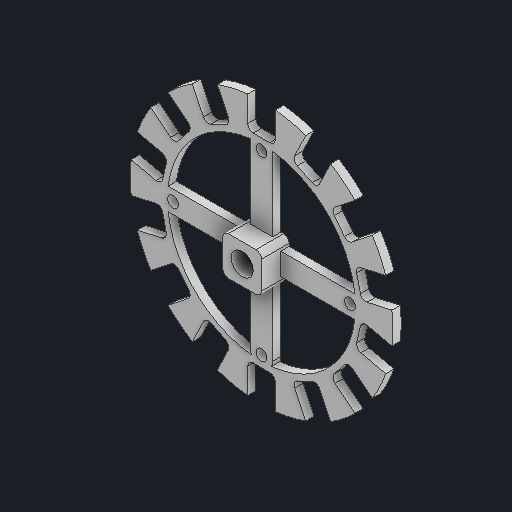
# Autodesk Inventor part: OmniFrame_A
Saved by Autodesk Inventor 2024.2 (Build 282272000, 272)
## iProperties
Created: 2023-12-20
Part Number: OmniFrame_A
Material: 一般
Document SubType Name: Modeling
Designer: Hanaoka
Density: 1 g/cm^3
Appearance: 既定
Author: Hanaoka
Autodesk Inventor part; units mm, degrees
ref_plane "YZ Plane" through (0, 0, 0) normal (1, 0, 0) x (0, 1, 0)
ref_plane "XZ Plane" through (0, 0, 0) normal (0, 1, 0) x (-1, 0, 0)
ref_plane "XY Plane" through (0, 0, 0) normal (0, 0, 1) x (1, 0, 0)
derived "OmniFrame_B.ipt"
sketch "スケッチ1" plane through (0, 0, 0) normal (0, 0, 1) x (1, 0, 0)
  circle A0 centre (0, 0) radius 25 construction
  line L0 (-2.5, 24.8747) -> (-2.5, 19)
  line L1 (-1.5, 18) -> (1.5, 18)
  line L2 (2.5, 19) -> (2.5, 24.8747)
  line L3 (0, 25) -> (0, 18) construction
  line L4 (-2.5, 23.025) -> (-3, 23.025)
  line L5 (-4, 22.025) -> (-4, 21.975)
  line L6 (-3, 20.975) -> (-2.5, 20.975)
  line L7 (2.5, 23.025) -> (3, 23.025)
  line L8 (4, 22.025) -> (4, 21.975)
  line L9 (3, 20.975) -> (2.5, 20.975)
  arc A1 (-3, 23.025) -> (-4, 22.025) centre (-3, 22.025) ccw
  arc A2 (-4, 21.975) -> (-3, 20.975) centre (-3, 21.975) ccw
  arc A3 (4, 22.025) -> (3, 23.025) centre (3, 22.025) ccw
  arc A4 (3, 20.975) -> (4, 21.975) centre (3, 21.975) ccw
  arc A5 (-2.5, 19) -> (-1.5, 18) centre (-1.5, 19) ccw
  arc A6 (1.5, 18) -> (2.5, 19) centre (1.5, 19) ccw
  arc A7 (-10.4962, 16.0337) -> (-9.1614, 15.5666) centre (-9.5952, 16.4676) ccw
  arc A8 (-6.4585, 16.8683) -> (-5.9914, 18.2031) centre (-6.8923, 17.7692) ccw
  line L10 (-9.1614, 15.5666) -> (-6.4585, 16.8683)
  line L11 (-6.3978, 20.1995) -> (-6.8483, 19.9825)
  arc A9 (-6.3978, 20.1995) -> (-5.9307, 21.5343) centre (-6.8317, 21.1004) ccw
  line L12 (-5.9524, 21.5794) -> (-5.9307, 21.5343)
  arc A10 (-5.9524, 21.5794) -> (-7.2873, 22.0465) centre (-6.8534, 21.1455) ccw
  line L13 (-7.7378, 21.8295) -> (-7.2873, 22.0465)
  line L14 (-11.8036, 17.5962) -> (-11.3531, 17.8131)
  line L15 (-5.9914, 18.2031) -> (-8.5403, 23.496)
  line L16 (-10.8471, 22.5242) -> (-7.8099, 16.2174) construction
  line L17 (-13.0451, 21.3266) -> (-10.4962, 16.0337)
  arc A11 (-13.1385, 18.0633) -> (-11.8036, 17.5962) centre (-12.2375, 18.4971) ccw
  line L18 (-12.2426, 19.6601) -> (-12.6931, 19.4432)
  line L19 (-13.1602, 18.1083) -> (-13.1385, 18.0633)
  arc A12 (-12.6931, 19.4432) -> (-13.1602, 18.1083) centre (-12.2592, 18.5422) ccw
  arc A13 (-16.4135, 9.8917) -> (-15.0082, 10.0501) centre (-15.79, 10.6736) ccw
  arc A14 (-13.1377, 12.3956) -> (-13.2961, 13.8009) centre (-13.9196, 13.0191) ccw
  line L20 (-15.0082, 10.0501) -> (-13.1377, 12.3956)
  line L21 (-14.5284, 15.4232) -> (-14.8402, 15.0323)
  arc A15 (-14.5284, 15.4232) -> (-14.6868, 16.8285) centre (-15.3103, 16.0467) ccw
  line L22 (-14.7259, 16.8597) -> (-14.6868, 16.8285)
  arc A16 (-14.7259, 16.8597) -> (-16.1312, 16.7013) centre (-15.3494, 16.0779) ccw
  line L23 (-16.4429, 16.3104) -> (-16.1312, 16.7013)
  line L24 (-18.2694, 10.7322) -> (-17.9576, 11.1231)
  line L25 (-13.2961, 13.8009) -> (-17.8891, 17.4637)
  line L26 (-19.5458, 15.5872) -> (-14.073, 11.2228) construction
  line L27 (-21.0065, 13.5545) -> (-16.4135, 9.8917)
  arc A17 (-19.6747, 10.5739) -> (-18.2694, 10.7322) centre (-19.0512, 11.3557) ccw
  line L28 (-19.5604, 12.4013) -> (-19.8721, 12.0104)
  line L29 (-19.7138, 10.605) -> (-19.6747, 10.5739)
  arc A18 (-19.8721, 12.0104) -> (-19.7138, 10.605) centre (-19.0903, 11.3869) ccw
  arc A19 (-19.0799, 1.7906) -> (-17.8825, 2.543) centre (-18.8574, 2.7655) ccw
  arc A20 (-17.2149, 5.4678) -> (-17.9673, 6.6652) centre (-18.1898, 5.6903) ccw
  line L30 (-17.8825, 2.543) -> (-17.2149, 5.4678)
  line L31 (-19.7816, 7.5922) -> (-19.8928, 7.1047)
  arc A21 (-19.7816, 7.5922) -> (-20.534, 8.7896) centre (-20.7565, 7.8147) ccw
  line L32 (-20.5827, 8.8007) -> (-20.534, 8.7896)
  arc A22 (-20.5827, 8.8007) -> (-21.7802, 8.0483) centre (-20.8052, 7.8258) ccw
  line L33 (-21.8914, 7.5609) -> (-21.7802, 8.0483)
  line L34 (-21.1167, 1.7426) -> (-21.0054, 2.2301)
  line L35 (-17.9673, 6.6652) -> (-23.6947, 7.9725)
  line L36 (-24.3732, 5.563) -> (-17.5487, 4.0054) construction
  line L37 (-24.8073, 3.0978) -> (-19.0799, 1.7906)
  arc A23 (-22.3141, 0.9902) -> (-21.1167, 1.7426) centre (-22.0916, 1.9651) ccw
  line L38 (-23.004, 2.6862) -> (-23.1153, 2.1988)
  line L39 (-22.3629, 1.0013) -> (-22.3141, 0.9902)
  arc A24 (-23.1153, 2.1988) -> (-22.3629, 1.0013) centre (-22.1404, 1.9762) ccw
  arc A25 (-17.9673, -6.6652) -> (-17.2149, -5.4678) centre (-18.1898, -5.6903) ccw
  arc A26 (-17.8825, -2.543) -> (-19.0799, -1.7906) centre (-18.8574, -2.7655) ccw
  line L40 (-17.2149, -5.4678) -> (-17.8825, -2.543)
  line L41 (-21.1167, -1.7426) -> (-21.0054, -2.2301)
  arc A27 (-21.1167, -1.7426) -> (-22.3141, -0.9902) centre (-22.0916, -1.9651) ccw
  line L42 (-22.3629, -1.0013) -> (-22.3141, -0.9902)
  arc A28 (-22.3629, -1.0013) -> (-23.1153, -2.1988) centre (-22.1404, -1.9762) ccw
  line L43 (-23.004, -2.6862) -> (-23.1153, -2.1988)
  line L44 (-19.7816, -7.5922) -> (-19.8928, -7.1047)
  line L45 (-19.0799, -1.7906) -> (-24.8073, -3.0978)
  line L46 (-24.3732, -5.563) -> (-17.5487, -4.0054) construction
  line L47 (-23.6947, -7.9725) -> (-17.9673, -6.6652)
  arc A29 (-20.534, -8.7896) -> (-19.7816, -7.5922) centre (-20.7565, -7.8147) ccw
  line L48 (-21.8914, -7.5609) -> (-21.7802, -8.0483)
  line L49 (-20.5827, -8.8007) -> (-20.534, -8.7896)
  arc A30 (-21.7802, -8.0483) -> (-20.5827, -8.8007) centre (-20.8052, -7.8258) ccw
  arc A31 (-13.2961, -13.8009) -> (-13.1377, -12.3956) centre (-13.9196, -13.0191) ccw
  arc A32 (-15.0082, -10.0501) -> (-16.4135, -9.8917) centre (-15.79, -10.6736) ccw
  line L50 (-13.1377, -12.3956) -> (-15.0082, -10.0501)
  line L51 (-18.2694, -10.7322) -> (-17.9576, -11.1231)
  arc A33 (-18.2694, -10.7322) -> (-19.6747, -10.5739) centre (-19.0512, -11.3557) ccw
  line L52 (-19.7138, -10.605) -> (-19.6747, -10.5739)
  arc A34 (-19.7138, -10.605) -> (-19.8721, -12.0104) centre (-19.0903, -11.3869) ccw
  line L53 (-19.5604, -12.4013) -> (-19.8721, -12.0104)
  line L54 (-14.5284, -15.4232) -> (-14.8402, -15.0323)
  line L55 (-16.4135, -9.8917) -> (-21.0065, -13.5545)
  line L56 (-19.5458, -15.5872) -> (-14.073, -11.2228) construction
  line L57 (-17.8891, -17.4637) -> (-13.2961, -13.8009)
  arc A35 (-14.6868, -16.8285) -> (-14.5284, -15.4232) centre (-15.3103, -16.0467) ccw
  line L58 (-16.4429, -16.3104) -> (-16.1312, -16.7013)
  line L59 (-14.7259, -16.8597) -> (-14.6868, -16.8285)
  arc A36 (-16.1312, -16.7013) -> (-14.7259, -16.8597) centre (-15.3494, -16.0779) ccw
  arc A37 (-5.9914, -18.2031) -> (-6.4585, -16.8683) centre (-6.8923, -17.7692) ccw
  arc A38 (-9.1614, -15.5666) -> (-10.4962, -16.0337) centre (-9.5952, -16.4676) ccw
  line L60 (-6.4585, -16.8683) -> (-9.1614, -15.5666)
  line L61 (-11.8036, -17.5962) -> (-11.3531, -17.8131)
  arc A39 (-11.8036, -17.5962) -> (-13.1385, -18.0633) centre (-12.2375, -18.4971) ccw
  line L62 (-13.1602, -18.1083) -> (-13.1385, -18.0633)
  arc A40 (-13.1602, -18.1083) -> (-12.6931, -19.4432) centre (-12.2592, -18.5422) ccw
  line L63 (-12.2426, -19.6601) -> (-12.6931, -19.4432)
  line L64 (-6.3978, -20.1995) -> (-6.8483, -19.9825)
  line L65 (-10.4962, -16.0337) -> (-13.0451, -21.3266)
  line L66 (-10.8471, -22.5242) -> (-7.8099, -16.2174) construction
  line L67 (-8.5403, -23.496) -> (-5.9914, -18.2031)
  arc A41 (-5.9307, -21.5343) -> (-6.3978, -20.1995) centre (-6.8317, -21.1004) ccw
  line L68 (-7.7378, -21.8295) -> (-7.2873, -22.0465)
  line L69 (-5.9524, -21.5794) -> (-5.9307, -21.5343)
  arc A42 (-7.2873, -22.0465) -> (-5.9524, -21.5794) centre (-6.8534, -21.1455) ccw
  arc A43 (2.5, -19) -> (1.5, -18) centre (1.5, -19) ccw
  arc A44 (-1.5, -18) -> (-2.5, -19) centre (-1.5, -19) ccw
  line L70 (1.5, -18) -> (-1.5, -18)
  line L71 (-3, -20.975) -> (-2.5, -20.975)
  arc A45 (-3, -20.975) -> (-4, -21.975) centre (-3, -21.975) ccw
  line L72 (-4, -22.025) -> (-4, -21.975)
  arc A46 (-4, -22.025) -> (-3, -23.025) centre (-3, -22.025) ccw
  line L73 (-2.5, -23.025) -> (-3, -23.025)
  line L74 (3, -20.975) -> (2.5, -20.975)
  line L75 (-2.5, -19) -> (-2.5, -24.8747)
  line L76 (0, -25) -> (0, -18) construction
  line L77 (2.5, -24.8747) -> (2.5, -19)
  arc A47 (4, -21.975) -> (3, -20.975) centre (3, -21.975) ccw
  line L78 (2.5, -23.025) -> (3, -23.025)
  line L79 (4, -22.025) -> (4, -21.975)
  arc A48 (3, -23.025) -> (4, -22.025) centre (3, -22.025) ccw
  arc A49 (10.4962, -16.0337) -> (9.1614, -15.5666) centre (9.5952, -16.4676) ccw
  arc A50 (6.4585, -16.8683) -> (5.9914, -18.2031) centre (6.8923, -17.7692) ccw
  line L80 (9.1614, -15.5666) -> (6.4585, -16.8683)
  line L81 (6.3978, -20.1995) -> (6.8483, -19.9825)
  arc A51 (6.3978, -20.1995) -> (5.9307, -21.5343) centre (6.8317, -21.1004) ccw
  line L82 (5.9524, -21.5794) -> (5.9307, -21.5343)
  arc A52 (5.9524, -21.5794) -> (7.2873, -22.0465) centre (6.8534, -21.1455) ccw
  line L83 (7.7378, -21.8295) -> (7.2873, -22.0465)
  line L84 (11.8036, -17.5962) -> (11.3531, -17.8131)
  line L85 (5.9914, -18.2031) -> (8.5403, -23.496)
  line L86 (10.8471, -22.5242) -> (7.8099, -16.2174) construction
  line L87 (13.0451, -21.3266) -> (10.4962, -16.0337)
  arc A53 (13.1385, -18.0633) -> (11.8036, -17.5962) centre (12.2375, -18.4971) ccw
  line L88 (12.2426, -19.6601) -> (12.6931, -19.4432)
  line L89 (13.1602, -18.1083) -> (13.1385, -18.0633)
  arc A54 (12.6931, -19.4432) -> (13.1602, -18.1083) centre (12.2592, -18.5422) ccw
  arc A55 (16.4135, -9.8917) -> (15.0082, -10.0501) centre (15.79, -10.6736) ccw
  arc A56 (13.1377, -12.3956) -> (13.2961, -13.8009) centre (13.9196, -13.0191) ccw
  line L90 (15.0082, -10.0501) -> (13.1377, -12.3956)
  line L91 (14.5284, -15.4232) -> (14.8402, -15.0323)
  arc A57 (14.5284, -15.4232) -> (14.6868, -16.8285) centre (15.3103, -16.0467) ccw
  line L92 (14.7259, -16.8597) -> (14.6868, -16.8285)
  arc A58 (14.7259, -16.8597) -> (16.1312, -16.7013) centre (15.3494, -16.0779) ccw
  line L93 (16.4429, -16.3104) -> (16.1312, -16.7013)
  line L94 (18.2694, -10.7322) -> (17.9576, -11.1231)
  line L95 (13.2961, -13.8009) -> (17.8891, -17.4637)
  line L96 (19.5458, -15.5872) -> (14.073, -11.2228) construction
  line L97 (21.0065, -13.5545) -> (16.4135, -9.8917)
  arc A59 (19.6747, -10.5739) -> (18.2694, -10.7322) centre (19.0512, -11.3557) ccw
  line L98 (19.5604, -12.4013) -> (19.8721, -12.0104)
  line L99 (19.7138, -10.605) -> (19.6747, -10.5739)
  arc A60 (19.8721, -12.0104) -> (19.7138, -10.605) centre (19.0903, -11.3869) ccw
  arc A61 (19.0799, -1.7906) -> (17.8825, -2.543) centre (18.8574, -2.7655) ccw
  arc A62 (17.2149, -5.4678) -> (17.9673, -6.6652) centre (18.1898, -5.6903) ccw
  line L100 (17.8825, -2.543) -> (17.2149, -5.4678)
  line L101 (19.7816, -7.5922) -> (19.8928, -7.1047)
  arc A63 (19.7816, -7.5922) -> (20.534, -8.7896) centre (20.7565, -7.8147) ccw
  line L102 (20.5827, -8.8007) -> (20.534, -8.7896)
  arc A64 (20.5827, -8.8007) -> (21.7802, -8.0483) centre (20.8052, -7.8258) ccw
  line L103 (21.8914, -7.5609) -> (21.7802, -8.0483)
  line L104 (21.1167, -1.7426) -> (21.0054, -2.2301)
  line L105 (17.9673, -6.6652) -> (23.6947, -7.9725)
  line L106 (24.3732, -5.563) -> (17.5487, -4.0054) construction
  line L107 (24.8073, -3.0978) -> (19.0799, -1.7906)
  arc A65 (22.3141, -0.9902) -> (21.1167, -1.7426) centre (22.0916, -1.9651) ccw
  line L108 (23.004, -2.6862) -> (23.1153, -2.1988)
  line L109 (22.3629, -1.0013) -> (22.3141, -0.9902)
  arc A66 (23.1153, -2.1988) -> (22.3629, -1.0013) centre (22.1404, -1.9762) ccw
  arc A67 (17.9673, 6.6652) -> (17.2149, 5.4678) centre (18.1898, 5.6903) ccw
  arc A68 (17.8825, 2.543) -> (19.0799, 1.7906) centre (18.8574, 2.7655) ccw
  line L110 (17.2149, 5.4678) -> (17.8825, 2.543)
  line L111 (21.1167, 1.7426) -> (21.0054, 2.2301)
  arc A69 (21.1167, 1.7426) -> (22.3141, 0.9902) centre (22.0916, 1.9651) ccw
  line L112 (22.3629, 1.0013) -> (22.3141, 0.9902)
  arc A70 (22.3629, 1.0013) -> (23.1153, 2.1988) centre (22.1404, 1.9762) ccw
  line L113 (23.004, 2.6862) -> (23.1153, 2.1988)
  line L114 (19.7816, 7.5922) -> (19.8928, 7.1047)
  line L115 (19.0799, 1.7906) -> (24.8073, 3.0978)
  line L116 (24.3732, 5.563) -> (17.5487, 4.0054) construction
  line L117 (23.6947, 7.9725) -> (17.9673, 6.6652)
  arc A71 (20.534, 8.7896) -> (19.7816, 7.5922) centre (20.7565, 7.8147) ccw
  line L118 (21.8914, 7.5609) -> (21.7802, 8.0483)
  line L119 (20.5827, 8.8007) -> (20.534, 8.7896)
  arc A72 (21.7802, 8.0483) -> (20.5827, 8.8007) centre (20.8052, 7.8258) ccw
  arc A73 (13.2961, 13.8009) -> (13.1377, 12.3956) centre (13.9196, 13.0191) ccw
  arc A74 (15.0082, 10.0501) -> (16.4135, 9.8917) centre (15.79, 10.6736) ccw
  line L120 (13.1377, 12.3956) -> (15.0082, 10.0501)
  line L121 (18.2694, 10.7322) -> (17.9576, 11.1231)
  arc A75 (18.2694, 10.7322) -> (19.6747, 10.5739) centre (19.0512, 11.3557) ccw
  line L122 (19.7138, 10.605) -> (19.6747, 10.5739)
  arc A76 (19.7138, 10.605) -> (19.8721, 12.0104) centre (19.0903, 11.3869) ccw
  line L123 (19.5604, 12.4013) -> (19.8721, 12.0104)
  line L124 (14.5284, 15.4232) -> (14.8402, 15.0323)
  line L125 (16.4135, 9.8917) -> (21.0065, 13.5545)
  line L126 (19.5458, 15.5872) -> (14.073, 11.2228) construction
  line L127 (17.8891, 17.4637) -> (13.2961, 13.8009)
  arc A77 (14.6868, 16.8285) -> (14.5284, 15.4232) centre (15.3103, 16.0467) ccw
  line L128 (16.4429, 16.3104) -> (16.1312, 16.7013)
  line L129 (14.7259, 16.8597) -> (14.6868, 16.8285)
  arc A78 (16.1312, 16.7013) -> (14.7259, 16.8597) centre (15.3494, 16.0779) ccw
  arc A79 (5.9914, 18.2031) -> (6.4585, 16.8683) centre (6.8923, 17.7692) ccw
  arc A80 (9.1614, 15.5666) -> (10.4962, 16.0337) centre (9.5952, 16.4676) ccw
  line L130 (6.4585, 16.8683) -> (9.1614, 15.5666)
  line L131 (11.8036, 17.5962) -> (11.3531, 17.8131)
  arc A81 (11.8036, 17.5962) -> (13.1385, 18.0633) centre (12.2375, 18.4971) ccw
  line L132 (13.1602, 18.1083) -> (13.1385, 18.0633)
  arc A82 (13.1602, 18.1083) -> (12.6931, 19.4432) centre (12.2592, 18.5422) ccw
  line L133 (12.2426, 19.6601) -> (12.6931, 19.4432)
  line L134 (6.3978, 20.1995) -> (6.8483, 19.9825)
  line L135 (10.4962, 16.0337) -> (13.0451, 21.3266)
  line L136 (10.8471, 22.5242) -> (7.8099, 16.2174) construction
  line L137 (8.5403, 23.496) -> (5.9914, 18.2031)
  arc A83 (5.9307, 21.5343) -> (6.3978, 20.1995) centre (6.8317, 21.1004) ccw
  line L138 (7.7378, 21.8295) -> (7.2873, 22.0465)
  line L139 (5.9524, 21.5794) -> (5.9307, 21.5343)
  arc A84 (7.2873, 22.0465) -> (5.9524, 21.5794) centre (6.8534, 21.1455) ccw
  circle A85 centre (0, 0) radius 23.75
  circle A86 centre (0, 0) radius 17
  circle A87 centre (0, 0) radius 2
  line L140 (-2.5, -3.5) -> (2.5, -3.5)
  line L141 (3.5, -2.5) -> (3.5, 2.5)
  line L142 (2.5, 3.5) -> (-2.5, 3.5)
  line L143 (-3.5, 2.5) -> (-3.5, -2.5)
  line L144 (-3.5, -3.5) -> (3.5, 3.5) construction
  line L145 (3.5, -3.5) -> (-3.5, 3.5) construction
  arc A88 (-2.5, 3.5) -> (-3.5, 2.5) centre (-2.5, 2.5) ccw
  arc A89 (-3.5, -2.5) -> (-2.5, -3.5) centre (-2.5, -2.5) ccw
  arc A90 (2.5, -3.5) -> (3.5, -2.5) centre (2.5, -2.5) ccw
  arc A91 (3.5, 2.5) -> (2.5, 3.5) centre (2.5, 2.5) ccw
  line L146 (-2, 16.8819) -> (-2, 3.5)
  line L147 (2, 3.5) -> (2, 16.8819)
  circle A92 centre (0, 16) radius 1
  line L148 (0, -35) -> (0, 35)
  circle A93 centre (0, 16) radius 2
  circle A94 centre (-16, 0) radius 1
  line L149 (-3.5, 2) -> (-16.8819, 2)
  line L150 (-16.8819, -2) -> (-3.5, -2)
  circle A95 centre (0, -16) radius 1
  line L151 (-2, -3.5) -> (-2, -16.8819)
  line L152 (2, -16.8819) -> (2, -3.5)
  circle A96 centre (16, 0) radius 1
  line L153 (3.5, -2) -> (16.8819, -2)
  line L154 (16.8819, 2) -> (3.5, 2)
  circle A97 centre (-16, 0) radius 2
  circle A98 centre (0, -16) radius 2
  circle A99 centre (16, 0) radius 2
  point P0 (-2.5, 18)
  point P1 (2.5, 18)
  point P2 (4, 23.025)
  point P3 (4, 20.975)
  point P4 (-4, 22)
  point P5 (-10.0623, 15.1327)
  point P6 (-5.5575, 17.3021)
  point P7 (-5.4968, 20.6334)
  point P8 (-6.3863, 22.4803)
  point P9 (-13.1493, 18.0858)
  point P10 (-15.6317, 9.2682)
  point P11 (-12.5142, 13.1774)
  point P12 (-13.905, 16.205)
  point P13 (-15.5077, 17.4832)
  point P14 (-19.6943, 10.5894)
  point P15 (-18.105, 1.5681)
  point P16 (-16.9924, 6.4427)
  point P17 (-19.559, 8.5671)
  point P18 (-21.5576, 9.0233)
  point P19 (-22.3385, 0.9957)
  point P20 (-16.9924, -6.4427)
  point P21 (-18.105, -1.5681)
  point P22 (-21.3392, -0.7677)
  point P23 (-23.3378, -1.2238)
  point P24 (-20.5583, -8.7952)
  point P25 (-12.5142, -13.1774)
  point P26 (-15.6317, -9.2682)
  point P27 (-18.8929, -9.9504)
  point P28 (-20.4956, -11.2285)
  point P29 (-14.7063, -16.8441)
  point P30 (-5.5575, -17.3021)
  point P31 (-10.0623, -15.1327)
  point P32 (-12.7046, -17.1623)
  point P33 (-13.594, -19.0093)
  point P34 (-5.9416, -21.5569)
  point P35 (2.5, -18)
  point P36 (-2.5, -18)
  point P37 (-4, -20.975)
  point P38 (-4, -23.025)
  point P39 (4, -22)
  point P40 (10.0623, -15.1327)
  point P41 (5.5575, -17.3021)
  point P42 (5.4968, -20.6334)
  point P43 (6.3863, -22.4803)
  point P44 (13.1493, -18.0858)
  point P45 (15.6317, -9.2682)
  point P46 (12.5142, -13.1774)
  point P47 (13.905, -16.205)
  point P48 (15.5077, -17.4832)
  point P49 (19.6943, -10.5894)
  point P50 (18.105, -1.5681)
  point P51 (16.9924, -6.4427)
  point P52 (19.559, -8.5671)
  point P53 (21.5576, -9.0233)
  point P54 (22.3385, -0.9957)
  point P55 (16.9924, 6.4427)
  point P56 (18.105, 1.5681)
  point P57 (21.3392, 0.7677)
  point P58 (23.3378, 1.2238)
  point P59 (20.5583, 8.7952)
  point P60 (12.5142, 13.1774)
  point P61 (15.6317, 9.2682)
  point P62 (18.8929, 9.9504)
  point P63 (20.4956, 11.2285)
  point P64 (14.7063, 16.8441)
  point P65 (5.5575, 17.3021)
  point P66 (10.0623, 15.1327)
  point P67 (12.7046, 17.1623)
  point P68 (13.594, 19.0093)
  point P69 (5.9416, 21.5569)
  point P70 (-1.7829, -16.9063)
  point P71 (-16.9063, -1.7829)
  point P72 (-16.9063, 1.7829)
  point P73 (-1.7829, 16.9063)
  point P74 (0, 18)
  point P75 (-2.5, 23.6181)
  point P76 (-7.9951, 22.3638)
  point P77 (-12.4999, 20.1944)
  point P78 (-16.9066, 16.6802)
  point P79 (-20.0241, 12.771)
  point P80 (-22.4696, 7.6928)
  point P81 (-23.5822, 2.8182)
  point P82 (-23.5822, -2.8182)
  point P83 (-22.4696, -7.6928)
  point P84 (-20.0241, -12.771)
  point P85 (-16.9066, -16.6802)
  point P86 (-12.4999, -20.1944)
  point P87 (-7.9951, -22.3638)
  point P88 (-2.5, -23.6181)
  point P89 (2.5, -23.6181)
  point P90 (7.9951, -22.3638)
  point P91 (12.4999, -20.1944)
  point P92 (16.9066, -16.6802)
  point P93 (20.0241, -12.771)
  point P94 (22.4696, -7.6928)
  point P95 (23.5822, -2.8182)
  point P96 (23.5822, 2.8182)
  point P97 (22.4696, 7.6928)
  point P98 (20.0241, 12.771)
  point P99 (16.9066, 16.6802)
  point P100 (12.4999, 20.1944)
  point P101 (7.9951, 22.3638)
  point P102 (2.5, 23.6181)
  point P103 (1.7829, 16.9063)
  point P104 (16.9063, 1.7829)
  point P105 (16.9063, -1.7829)
  point P106 (1.7829, -16.9063)
  point P107 (2, -16)
  point P108 (2, -3.5)
  point P109 (-2, -16)
  point P110 (-16.8819, 2)
  point P111 (-16.8819, -2)
  point P112 (-3.5, -2)
  point P113 (16.8819, -2)
  point P114 (3.5, 2)
extrude "押し出し1" add sketch "スケッチ1" along normal blind 1.5 contours L4 A1 L5 A2 L6 L0 A5 L1 A93 A86 A97 A98 L70 A44 L75 L71 A45 L72 A46 L73 A85 L67 L68 A42 L69 A41 L64 A37 L60 A38 L65 L61 A39 L62 A40 L63 L57 L58 A36 L59 A35 L54 A31 L50 A32 L55 L51 A33 L52 A34 L53 L47 L48 A30 L49 A29 L44 A25 L40 A26 L45 L41 A27 L42 A28 L43 L37 L38 A24 L39 A23 L34 A19 L30 A20 L35 L31 A21 L32 A22 L33 L27 L28 A18 L29 A17 L24 A13 L20 A14 L25 L21 A15 L22 A16 L23 L17 L18 A12 L19 A11 L14 A7 L10 A8 L15 L11 A9 L12 A10 L13 | L0 L6 A2 L5 A1 L4 | A85 L137 L138 A84 L139 A83 L134 A79 L130 A80 L135 L131 A81 L132 A82 L133 L127 L128 A78 L129 A77 L124 A73 L120 A74 L125 L121 A75 L122 A76 L123 L117 L118 A72 L119 A71 L114 A67 L110 A68 L115 L111 A69 L112 A70 L113 L107 L108 A66 L109 A65 L104 A61 L100 A62 L105 L101 A63 L102 A64 L103 L97 L98 A60 L99 A59 L94 A55 L90 A56 L95 L91 A57 L92 A58 L93 L87 L88 A54 L89 A53 L84 A49 L80 A50 L85 L81 A51 L82 A52 L83 L77 L78 A48 L79 A47 L74 A43 L70 A98 A86 A99 A93 L1 A6 L2 L9 A4 L8 A3 L7 | A93 A86 L148 | L148 A86 A93 | L13 A10 L12 A9 L11 L15 | L7 A3 L8 A4 L9 L2 | A92 L148 A93 A86 | A86 A93 L148 A92 | A86 L147 A93 | A93 L146 A86 | L17 L14 A11 L19 A12 L18 | L137 L134 A83 L139 A84 L138 | L147 L142 L148 A93 | A93 L148 L142 L146 | L23 A16 L22 A15 L21 L25 | L133 A82 L132 A81 L131 L135 | A86 A99 L154 | L142 A91 L141 A90 L140 L148 A87 | L149 A97 A86 | L142 L148 A87 L140 A89 L143 A88 | L27 L24 A17 L29 A18 L28 | L127 L124 A77 L129 A78 L128 | A99 A86 | A86 A99 | A99 L153 L141 L154 | A97 A86 | A86 A97 | L149 L143 L150 A97 | L33 A22 L32 A21 L31 L35 | L123 A76 L122 A75 L121 L125 | A99 A86 L153 | A97 L150 A86 | L37 L34 A23 L39 A24 L38 | L117 L114 A71 L119 A72 L118 | L43 A28 L42 A27 L41 L45 | L113 A70 L112 A69 L111 L115 | L148 A98 L151 L140 | L140 L152 A98 L148 | L47 L44 A29 L49 A30 L48 | A98 A86 A95 L148 | L148 A95 A86 A98 | A98 L148 A86 | A86 L148 A98 | L53 A34 L52 A33 L51 L55 | L107 L104 A65 L109 A66 L108 | L57 L54 A35 L59 A36 L58 | L103 A64 L102 A63 L101 L105 | L63 A40 L62 A39 L61 L65 | L97 L94 A59 L99 A60 L98 | L67 L64 A41 L69 A42 L68 | L93 A58 L92 A57 L91 L95 | L74 A47 L79 A48 L78 L77 | L75 L73 A46 L72 A45 L71 | L87 L84 A53 L89 A54 L88 | L83 A52 L82 A51 L81 L85
extrude "押し出し2" add sketch "スケッチ1" along normal blind 5 contours L142 A91 L141 A90 L140 L148 A87 | L142 L148 A87 L140 A89 L143 A88
